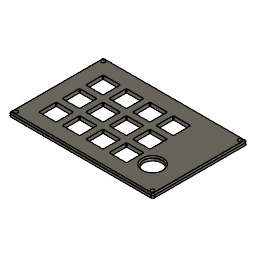
pablo_macro_case_lid (Autodesk Fusion 360 design; units mm, degrees)
part number: 2026-03-05-21-03-19-459
Autodesk Fusion 360 part; units mm, degrees
sketch "plate-2026-03-05T18_28_15.155Z" plane through (0, 0, 0) normal (0, 0, 1) x (1, 0, 0)
  line L0 (3.025, -2.525) -> (16.025, -2.525)
  line L1 (3.025, -16.525) -> (16.025, -16.525)
  line L2 (2.525, -3.025) -> (2.525, -16.025)
  line L3 (16.525, -3.025) -> (16.525, -16.025)
  arc A0 (3.025, -2.525) -> (2.525, -3.025) centre (3.025, -3.025) ccw
  arc A1 (16.525, -3.025) -> (16.025, -2.525) centre (16.025, -3.025) ccw
  arc A2 (2.525, -16.025) -> (3.025, -16.525) centre (3.025, -16.025) ccw
  arc A3 (16.025, -16.525) -> (16.525, -16.025) centre (16.025, -16.025) ccw
  line L4 (22.075, -2.525) -> (35.075, -2.525)
  line L5 (22.075, -16.525) -> (35.075, -16.525)
  line L6 (21.575, -3.025) -> (21.575, -16.025)
  line L7 (35.575, -3.025) -> (35.575, -16.025)
  arc A4 (22.075, -2.525) -> (21.575, -3.025) centre (22.075, -3.025) ccw
  arc A5 (35.575, -3.025) -> (35.075, -2.525) centre (35.075, -3.025) ccw
  arc A6 (21.575, -16.025) -> (22.075, -16.525) centre (22.075, -16.025) ccw
  arc A7 (35.075, -16.525) -> (35.575, -16.025) centre (35.075, -16.025) ccw
  line L8 (41.125, -2.525) -> (54.125, -2.525)
  line L9 (41.125, -16.525) -> (54.125, -16.525)
  line L10 (40.625, -3.025) -> (40.625, -16.025)
  line L11 (54.625, -3.025) -> (54.625, -16.025)
  arc A8 (41.125, -2.525) -> (40.625, -3.025) centre (41.125, -3.025) ccw
  arc A9 (54.625, -3.025) -> (54.125, -2.525) centre (54.125, -3.025) ccw
  arc A10 (40.625, -16.025) -> (41.125, -16.525) centre (41.125, -16.025) ccw
  arc A11 (54.125, -16.525) -> (54.625, -16.025) centre (54.125, -16.025) ccw
  line L12 (60.175, -2.525) -> (73.175, -2.525)
  line L13 (60.175, -16.525) -> (73.175, -16.525)
  line L14 (59.675, -3.025) -> (59.675, -16.025)
  line L15 (73.675, -3.025) -> (73.675, -16.025)
  arc A12 (60.175, -2.525) -> (59.675, -3.025) centre (60.175, -3.025) ccw
  arc A13 (73.675, -3.025) -> (73.175, -2.525) centre (73.175, -3.025) ccw
  arc A14 (59.675, -16.025) -> (60.175, -16.525) centre (60.175, -16.025) ccw
  arc A15 (73.175, -16.525) -> (73.675, -16.025) centre (73.175, -16.025) ccw
  line L16 (3.025, -21.575) -> (16.025, -21.575)
  line L17 (3.025, -35.575) -> (16.025, -35.575)
  line L18 (2.525, -22.075) -> (2.525, -35.075)
  line L19 (16.525, -22.075) -> (16.525, -35.075)
  arc A16 (3.025, -21.575) -> (2.525, -22.075) centre (3.025, -22.075) ccw
  arc A17 (16.525, -22.075) -> (16.025, -21.575) centre (16.025, -22.075) ccw
  arc A18 (2.525, -35.075) -> (3.025, -35.575) centre (3.025, -35.075) ccw
  arc A19 (16.025, -35.575) -> (16.525, -35.075) centre (16.025, -35.075) ccw
  line L20 (22.075, -21.575) -> (35.075, -21.575)
  line L21 (22.075, -35.575) -> (35.075, -35.575)
  line L22 (21.575, -22.075) -> (21.575, -35.075)
  line L23 (35.575, -22.075) -> (35.575, -35.075)
  arc A20 (22.075, -21.575) -> (21.575, -22.075) centre (22.075, -22.075) ccw
  arc A21 (35.575, -22.075) -> (35.075, -21.575) centre (35.075, -22.075) ccw
  arc A22 (21.575, -35.075) -> (22.075, -35.575) centre (22.075, -35.075) ccw
  arc A23 (35.075, -35.575) -> (35.575, -35.075) centre (35.075, -35.075) ccw
  line L24 (41.125, -21.575) -> (54.125, -21.575)
  line L25 (41.125, -35.575) -> (54.125, -35.575)
  line L26 (40.625, -22.075) -> (40.625, -35.075)
  line L27 (54.625, -22.075) -> (54.625, -35.075)
  arc A24 (41.125, -21.575) -> (40.625, -22.075) centre (41.125, -22.075) ccw
  arc A25 (54.625, -22.075) -> (54.125, -21.575) centre (54.125, -22.075) ccw
  arc A26 (40.625, -35.075) -> (41.125, -35.575) centre (41.125, -35.075) ccw
  arc A27 (54.125, -35.575) -> (54.625, -35.075) centre (54.125, -35.075) ccw
  line L28 (60.175, -21.575) -> (73.175, -21.575)
  line L29 (60.175, -35.575) -> (73.175, -35.575)
  line L30 (59.675, -22.075) -> (59.675, -35.075)
  line L31 (73.675, -22.075) -> (73.675, -35.075)
  arc A28 (60.175, -21.575) -> (59.675, -22.075) centre (60.175, -22.075) ccw
  arc A29 (73.675, -22.075) -> (73.175, -21.575) centre (73.175, -22.075) ccw
  arc A30 (59.675, -35.075) -> (60.175, -35.575) centre (60.175, -35.075) ccw
  arc A31 (73.175, -35.575) -> (73.675, -35.075) centre (73.175, -35.075) ccw
  line L32 (3.025, -40.625) -> (16.025, -40.625)
  line L33 (3.025, -54.625) -> (16.025, -54.625)
  line L34 (2.525, -41.125) -> (2.525, -54.125)
  line L35 (16.525, -41.125) -> (16.525, -54.125)
  arc A32 (3.025, -40.625) -> (2.525, -41.125) centre (3.025, -41.125) ccw
  arc A33 (16.525, -41.125) -> (16.025, -40.625) centre (16.025, -41.125) ccw
  arc A34 (2.525, -54.125) -> (3.025, -54.625) centre (3.025, -54.125) ccw
  arc A35 (16.025, -54.625) -> (16.525, -54.125) centre (16.025, -54.125) ccw
  line L36 (22.075, -40.625) -> (35.075, -40.625)
  line L37 (22.075, -54.625) -> (35.075, -54.625)
  line L38 (21.575, -41.125) -> (21.575, -54.125)
  line L39 (35.575, -41.125) -> (35.575, -54.125)
  arc A36 (22.075, -40.625) -> (21.575, -41.125) centre (22.075, -41.125) ccw
  arc A37 (35.575, -41.125) -> (35.075, -40.625) centre (35.075, -41.125) ccw
  arc A38 (21.575, -54.125) -> (22.075, -54.625) centre (22.075, -54.125) ccw
  arc A39 (35.075, -54.625) -> (35.575, -54.125) centre (35.075, -54.125) ccw
  line L40 (41.125, -40.625) -> (54.125, -40.625)
  line L41 (41.125, -54.625) -> (54.125, -54.625)
  line L42 (40.625, -41.125) -> (40.625, -54.125)
  line L43 (54.625, -41.125) -> (54.625, -54.125)
  arc A40 (41.125, -40.625) -> (40.625, -41.125) centre (41.125, -41.125) ccw
  arc A41 (54.625, -41.125) -> (54.125, -40.625) centre (54.125, -41.125) ccw
  arc A42 (40.625, -54.125) -> (41.125, -54.625) centre (41.125, -54.125) ccw
  arc A43 (54.125, -54.625) -> (54.625, -54.125) centre (54.125, -54.125) ccw
  line L44 (60.175, -40.625) -> (73.175, -40.625)
  line L45 (60.175, -54.625) -> (73.175, -54.625)
  line L46 (59.675, -41.125) -> (59.675, -54.125)
  line L47 (73.675, -41.125) -> (73.675, -54.125)
  arc A44 (60.175, -40.625) -> (59.675, -41.125) centre (60.175, -41.125) ccw
  arc A45 (73.675, -41.125) -> (73.175, -40.625) centre (73.175, -41.125) ccw
  arc A46 (59.675, -54.125) -> (60.175, -54.625) centre (60.175, -54.125) ccw
  arc A47 (73.175, -54.625) -> (73.675, -54.125) centre (73.175, -54.125) ccw
  line L48 (-10.075, 10.375) -> (106.925, 10.375)
  line L49 (106.925, 10.375) -> (106.925, -66.625)
  line L50 (106.925, -66.625) -> (-10.075, -66.625)
  line L51 (-10.075, -66.625) -> (-10.075, 10.375)
  circle A48 centre (85.425, -45.125) radius 7.5
  circle A49 centre (103.925, 7.375) radius 1.55
  circle A50 centre (-7.075, 7.375) radius 1.55
  circle A51 centre (-7.075, -63.625) radius 1.55
  circle A52 centre (103.925, -63.625) radius 1.55
  dimension "d1" = 117
  dimension "d2" = 77
  dimension "d3" = 12.6
  dimension "d4" = 12.9
  dimension "d5" = 15
  dimension "d6" = 21.5
  dimension "d7" = 21.5
  dimension "d8" = 3.1
  dimension "d9" = 3.1
  dimension "d10" = 3.1
  dimension "d11" = 3.1
  dimension "d12" = 3
  dimension "d13" = 3
  dimension "d14" = 3
  dimension "d15" = 3
  dimension "d16" = 3
  dimension "d17" = 3
  dimension "d18" = 3
  dimension "d19" = 3
  constraint horizontal L48
  constraint vertical L49
  constraint horizontal L50
  constraint vertical L51
  measures "d1" distance of L48.start L48.end
  measures "d2" distance of L48.start L50.end
  measures "d3" distance of L2 L51
  measures "d4" distance of L0 L48
  measures "d5" diameter of A48
  measures "d6" distance of L49 A48.centre
  measures "d7" distance of L50 A48.centre
  measures "d8" diameter of A49
  measures "d9" diameter of A50
  measures "d10" diameter of A51
  measures "d11" diameter of A52
  measures "d12" distance of L49 A52.centre
  measures "d13" distance of L50 A52.centre
  measures "d14" distance of L50 A51.centre
  measures "d15" distance of L51 A51.centre
  measures "d16" distance of L48 A50.centre
  measures "d17" distance of L51 A50.centre
  measures "d18" distance of L48 A49.centre
  measures "d19" distance of L49 A49.centre
extrude "Extrude1" add sketch "plate-2026-03-05T18_28_15.155Z" along normal blind 3
fillet "Fillet1" radius 1 1 edges at (78.4325, -42.4129, 3)
fillet "Fillet2" radius 1 4 edges at (48.425, -66.625, 3) (106.925, -28.125, 3) (48.425, 10.375, 3) (-10.075, -28.125, 3)
fillet "Fillet3" radius 1.5 8 edges at (106.925, -66.625, 1) (106.6321, -66.3321, 2.7071) (106.925, 10.375, 1) (106.6321, 10.0821, 2.7071) (-10.075, 10.375, 1) (-9.7821, 10.0821, 2.7071) (-10.075, -66.625, 1) (-9.7821, -66.3321, 2.7071)
